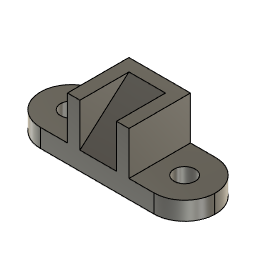
A2 (Autodesk Fusion 360 design; units mm, degrees)
Autodesk Fusion 360 part; units mm, degrees
note: some values were not read from the file. Set by a fixed rule: which sketch regions a step uses.
sketch "Sketch1" plane through (0, 0, 0) normal (0, 0, 1) x (1, 0, 0)
  line L0 (28.0323, 19.5121) -> (146.0361, 19.5121)
  line L1 (178.0242, -13.3588) -> (178.0327, -13.3589)
  line L2 (146.0457, -44.448) -> (28.0654, -44.448)
  line L3 (2.8649, 7.2735) -> (2.8643, 7.275)
  arc A0 (2.8649, 7.2735) -> (28.0654, -44.448) centre (28.0654, -12.448) ccw
  arc A1 (28.0323, 19.5121) -> (2.8643, 7.275) centre (28.0323, -12.4879) ccw
  arc A2 (178.0242, -13.3588) -> (146.0361, 19.5121) centre (146.0361, -12.4879) ccw
  arc A3 (146.0457, -44.448) -> (178.0327, -13.3589) centre (146.0457, -12.448) ccw
  circle A4 centre (28, -12.5) radius 11
  circle A5 centre (146, -12.5) radius 11
  line L4 (55.9792, 19.5121) -> (119.9792, 19.5121)
  line L5 (119.9792, 19.5121) -> (119.9792, -44.4879)
  line L6 (119.9792, -44.4879) -> (55.9792, -44.4879)
  line L7 (55.9792, -44.4879) -> (55.9792, 19.5121)
  point P0 (-1.9465, 19.5121)
  point P1 (176.0535, 19.5121)
  point P2 (0.3124, -44.448)
  dimension "d1" = 178
  dimension "d2" = 64
  dimension "d3" = 32
  dimension "d4" = 32
  dimension "d5" = 32
  dimension "d6" = 32
  dimension "d7" = 22
  dimension "d8" = 22
  dimension "d9" = 64
  dimension "d10" = 64
  constraint horizontal L0
  constraint horizontal L2
  constraint coincident P2 L2
  constraint tangent L2 A0
  constraint coincident P0 L0
  constraint coincident P0 L3
  constraint tangent L0 A1
  constraint coincident P1 L0
  constraint tangent L0 A2
  constraint tangent L2 A3
  constraint horizontal L4
  constraint vertical L5
  constraint horizontal L6
  constraint vertical L7
  constraint coincident L0 L4.start
  measures "d1" distance of P0 P1
  measures "d2" distance of P0 P2
  measures "d3" radius of A0
  measures "d4" radius of A1
  measures "d5" radius of A2
  measures "d6" radius of A3
  measures "d7" diameter of A4
  measures "d8" diameter of A5
  measures "d9" distance of L4.start L4.end
  measures "d10" distance of L4.start L6.end
extrude "Extrude1" add sketch "Sketch1" along normal blind 19 contours L0 L2 A0 A1 L7 | L0 L2 L4 L5 L7 | L0 L1 L2 A2 A3 L5
sketch "Sketch2" plane through (0, 0, 19) normal (0, 0, 1) x (-1, 0, 0)
  circle A0 centre (-146, 12.5) radius 11
  circle A1 centre (-28, 12.5) radius 11
  arc A2 (-28.0323, -19.5121) -> (-2.8643, -7.275) centre (-28.0323, 12.4879) ccw
  line L0 (-2.8643, -7.275) -> (-2.8649, -7.2735)
  arc A3 (-2.8649, -7.2735) -> (-28.0654, 44.448) centre (-28.0654, 12.448) ccw
  line L1 (-28.0654, 44.448) -> (-146.0457, 44.448)
  arc A4 (-146.0457, 44.448) -> (-178.0327, 13.3589) centre (-146.0457, 12.448) ccw
  line L2 (-178.0327, 13.3589) -> (-178.0242, 13.3588)
  arc A5 (-178.0242, 13.3588) -> (-146.0361, -19.5121) centre (-146.0361, 12.4879) ccw
  line L3 (-146.0361, -19.5121) -> (-28.0323, -19.5121)
  line L4 (-56.0201, -19.5121) -> (-120.0201, -19.5121)
  line L5 (-120.0201, -19.5121) -> (-120.0201, 44.4879)
  line L6 (-120.0201, 44.4879) -> (-56.0201, 44.4879)
  line L7 (-56.0201, 44.4879) -> (-56.0201, -19.5121)
  line L8 (-56.0201, 44.4879) -> (-69.0201, 44.4879)
  line L9 (-69.0201, 44.4879) -> (-69.0201, -6.5121)
  line L10 (-69.0201, -6.5121) -> (-107.0201, -6.5121)
  line L11 (-107.0201, -6.5121) -> (-107.0201, 44.4879)
  line L12 (-107.0201, 44.4879) -> (-120.0201, 44.4879)
  dimension "d13" = 64
  dimension "d14" = 64
  dimension "d15" = 13
  dimension "d16" = 51
  dimension "d17" = 38
  dimension "d18" = 51
  constraint horizontal L4
  constraint vertical L5
  constraint horizontal L6
  constraint vertical L7
  constraint coincident L3 L4.start
  constraint horizontal L8
  constraint perpendicular L6 L9
  constraint perpendicular L9 L10
  constraint perpendicular L1 L11
  measures "d13" distance of L4.start L4.end
  measures "d14" distance of L4.start L6.end
  measures "d15" distance of L6.end L8.end
  measures "d16" distance of L8.end L9.end
  measures "d17" distance of L9.end L10.end
  measures "d18" distance of L10.end L11.end
extrude "Extrude2" add sketch "Sketch2" along normal blind 45 contours L1 L3 L4 L5 L7 L9 L10 L11
sketch "Sketch3" plane through (69.0201, 0, 0) normal (1, 0, 0) x (0, 1, 0)
  line L0 (-44.448, 19) -> (6.5121, 19)
  line L1 (6.5121, 19) -> (6.5121, 64)
  line L2 (6.5121, 64) -> (-44.448, 64)
  line L3 (-44.448, 64) -> (-44.448, 19)
  line L4 (-44.448, 19) -> (6.552, 19)
  line L5 (6.552, 19) -> (6.5121, 64)
  line L6 (6.5121, 64) -> (-44.448, 19)
  dimension "d21" = 51
  constraint coincident L0.start L3.end
  constraint perpendicular L1 L4
  constraint coincident L1.end L2.start
  measures "d21" distance of L0.start L4.end
extrude "Extrude3" add sketch "Sketch3" along normal blind 38 contours L0 L1 L4 L6
named bodies: "A2"
